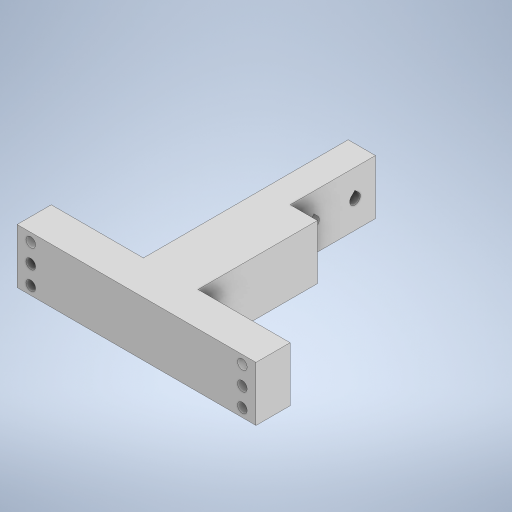
# Autodesk Inventor part: B1_head_T_twist
Saved by Autodesk Inventor 2023.1 (Build 271208000, 208)
## iProperties
Created: 2023-06-14
Part Number: B1_head_T_twist
Material: Generic
Document SubType Name: Modeling
Designer: zavrel
Density: 1 g/cm^3
Appearance: Default
Author: zavrel
Autodesk Inventor part; units mm, degrees
ref_plane "YZ Plane" through (0, 0, 0) normal (1, 0, 0) x (0, 1, 0)
ref_plane "XZ Plane" through (0, 0, 0) normal (0, 1, 0) x (-1, 0, 0)
ref_plane "XY Plane" through (0, 0, 0) normal (0, 0, 1) x (1, 0, 0)
sketch "Sketch1" plane through (0, 0, 0) normal (0, 1, 0) x (-1, 0, 0)
  line L0 (0, -29.3233) -> (8, -29.3233)
  line L1 (8, -29.3233) -> (8, 30.6767)
  line L2 (0, 0) -> (0, -29.3233) construction
  line L3 (0, -29.3233) -> (-8, -29.3233)
  line L4 (-8, -29.3233) -> (-8, 30.6767)
  line L5 (8, 30.6767) -> (35, 30.6767)
  line L6 (35, 30.6767) -> (35, 40.6767)
  line L7 (35, 40.6767) -> (2.1646, 40.6767)
  line L8 (2.1646, 40.6767) -> (0, 40.6767)
  line L9 (-8, 30.6767) -> (-35, 30.6767)
  line L10 (-35, 30.6767) -> (-35, 40.6767)
  line L11 (-35, 40.6767) -> (-2.1646, 40.6767)
  line L12 (-2.1646, 40.6767) -> (0, 40.6767)
  point P0 (4, -29.3233)
  point P1 (-4, -29.3233)
  dimension "d0" = 16
  dimension "d17" = 10
  dimension "d32" = 70
  dimension "d35" = 70
  constraints: 26 end point, 5 symmetric about line, 4 perpendicular, 2 midpoint, 1 collinear, 1 horizontal, 1 point on line, 1 vertical
  measures "d0" distance between parallel lines of L4 L1
  measures "d17" distance between parallel lines of L7 L5
  measures "d32" distance from line of point (-4, -29.323) L11
  measures "d35" distance between parallel lines of L10 L6
extrude "Extrusion1" add sketch "Sketch1" along normal blind 16
sketch "Sketch5" plane through (0.8354, 0, 40.6767) normal (0, 0, 1) x (1, 0, 0)
  line L0 (-35.8354, 0) -> (34.1646, 0) projected
  line L1 (-35.8354, 16) -> (34.1646, 16) projected
  line L2 (-35.8354, 0) -> (-35.8354, 16) projected
  line L3 (-35.8354, 0) -> (-35.8354, 16) construction
  line L4 (-35.8354, 8) -> (34.1646, 8) construction
  circle A0 centre (-31.8354, 13.5) radius 1.4
  circle A1 centre (-31.8354, 8) radius 1.4
  circle A2 centre (-31.8354, 2.5) radius 1.4
  line L5 (34.1646, 0) -> (34.1646, 16) projected
  line L6 (-35.8354, 16) -> (34.1646, 16) construction
  line L7 (-0.8354, 16) -> (-0.8354, 0) construction
  line L8 (-35.8354, 0) -> (34.1646, 0) projected
  circle A3 centre (30.1646, 13.5) radius 1.4
  circle A4 centre (30.1646, 8) radius 1.4
  circle A5 centre (30.1646, 2.5) radius 1.4
  dimension "d19" = 2.8
  dimension "d20" = 11
  dimension "d21" = 4
  constraints: 6 centre point, 4 end point, 4 midpoint, 4 symmetric about line, 1 equal radius, 1 point on line, 1 vertical alignment, 4 other
  measures "d19" diameter of A0
  measures "d20" distance of A2.centre A0.centre
  measures "d21" distance from line of L2 A1.centre
extrude "Extrusion8" cut sketch "Sketch5" against normal through all contours A0 | A1 | A2 | A3 | A4 | A5
sketch "Sketch9" plane through (8, 0, 30.6767) normal (1, 0, 0) x (0, 0, -1)
  line L0 (0, 0) -> (60, 0) projected
  line L1 (60, 0) -> (60, 16) projected
  line L2 (0, 16) -> (60, 16) projected
  line L3 (0, 0) -> (0, 16) projected
  line L4 (60, 0) -> (60, 16) construction
  line L5 (60, 8) -> (0, 8) construction
  line L6 (0, 0) -> (0, 16) construction
  circle A0 centre (54, 8) radius 1.55
  circle A1 centre (42, 8) radius 1.55
  line L7 (40.904, 9.096) -> (42, 10.192)
  line L8 (42, 10.192) -> (43.096, 9.096)
  line L9 (42, 8) -> (42, 13.728) construction
  line L10 (52.904, 9.096) -> (54, 10.192)
  line L11 (54, 10.192) -> (55.096, 9.096)
  point P0 (30.6767, 0)
  dimension "d36" = 12
  dimension "d37" = 3.1
  dimension "d38" = 6
  dimension "d47" = 90
  dimension "d48" = 90
  constraints: 12 end point, 3 point on line, 2 centre point, 2 midpoint, 2 point on circle, 2 tangent, 1 equal radius, 1 vertical
  measures "d36" distance of A0.centre L9.start
  measures "d37" diameter of A0
  measures "d38" distance from line of L1 A0.centre
  measures "d47" angle of L8 L7
  measures "d48" angle of L11 L10
extrude "Extrusion9" cut sketch "Sketch9" against normal through all contours A0 | A0 L10 L11 | A1 | A1 L7 L8
sketch "Sketch10" plane through (8, 0, 30.6767) normal (1, 0, 0) x (0, 0, -1)
  arc A0 (52.904, 9.096) -> (55.096, 9.096) centre (54, 8) ccw projected
  arc A1 (40.904, 9.096) -> (43.096, 9.096) centre (42, 8) ccw projected
  line L0 (0, 0) -> (60, 0) projected
  line L1 (60, 0) -> (60, 16) projected
  line L2 (0, 16) -> (60, 16) projected
  line L3 (0, 0) -> (0, 16) projected
  line L4 (60, 16) -> (35, 16)
  line L5 (35, 16) -> (35, 0)
  line L6 (35, 0) -> (60, 0)
  line L7 (60, 0) -> (60, 16)
  line L8 (54, 10.192) -> (55.096, 9.096) projected
  line L9 (52.904, 9.096) -> (54, 10.192) projected
  line L10 (42, 10.192) -> (43.096, 9.096) projected
  line L11 (40.904, 9.096) -> (42, 10.192) projected
  point P0 (30.6767, 0)
  dimension "d41" = 25
  constraints: 8 end point, 2 parallel, 1 horizontal, 1 perpendicular, 1 point on line
  measures "d41" distance between parallel lines of L1 L5
extrude "Extrusion10" cut sketch "Sketch10" against normal blind 8 contours L9 L8 A0 | L11 L10 A1 | L5 L2 L1 L0
sketch "Sketch11" plane through (-8, 0, -29.3233) normal (-1, 0, 0) x (0, 0, 1)
  arc A0 (4.904, 9.096) -> (7.096, 9.096) centre (6, 8) ccw projected
  arc A1 (16.904, 9.096) -> (19.096, 9.096) centre (18, 8) ccw projected
  line L0 (0, 0) -> (60, 0) projected
  line L1 (60, 0) -> (60, 16) projected
  line L2 (0, 16) -> (60, 16) projected
  line L3 (0, 0) -> (0, 16) projected
  circle A2 centre (18, 8) radius 3
  circle A3 centre (6, 8) radius 3
  line L4 (4.904, 9.096) -> (6, 10.192) projected
  line L5 (6, 10.192) -> (7.096, 9.096) projected
  line L6 (16.904, 9.096) -> (18, 10.192) projected
  line L7 (18, 10.192) -> (19.096, 9.096) projected
  line L8 (6, 8) -> (6, 12.7767) construction
  line L9 (6, 12.2426) -> (3.8787, 10.1213)
  line L10 (6, 12.2426) -> (8.1213, 10.1213)
  line L11 (18, 12.2426) -> (15.8787, 10.1213)
  line L12 (18, 12.2426) -> (20.1213, 10.1213)
  point P0 (29.3233, 0)
  dimension "d44" = 6
  dimension "d49" = 90
  dimension "d50" = 90
  constraints: 10 end point, 2 centre point, 2 coincident, 2 point on circle, 2 tangent, 1 equal radius, 1 point on line, 1 vertical
  measures "d44" diameter of A3
  measures "d49" angle of L10 L9
  measures "d50" angle of L12 L11
extrude "Extrusion11" cut sketch "Sketch11" against normal blind 3 contours L4 L5 A0 | L6 L7 A1 | A2 | A2 L11 L12 | A3 | A3 L9 L10
body "Solid1"
